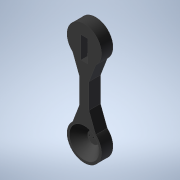
# Autodesk Inventor part: 1st-arm
Saved by Autodesk Inventor 2022 (Build 260153000, 153)
## iProperties
Created: 2022-02-04
Part Number: 1st-arm
Material: Generic
Document SubType Name: Modeling
Designer: Alexa
Density: 1 g/cm^3
Appearance: Default
Author: Alexa
Autodesk Inventor part; units mm, degrees
ref_plane "YZ Plane" through (0, 0, 0) normal (1, 0, 0) x (0, 1, 0)
ref_plane "XZ Plane" through (0, 0, 0) normal (0, 1, 0) x (-1, 0, 0)
ref_plane "XY Plane" through (0, 0, 0) normal (0, 0, 1) x (1, 0, 0)
sketch "Sketch1" plane through (0, 0, 0) normal (0, 0, 1) x (1, 0, 0)
  circle A0 centre (0, 0) radius 30
  line L0 (0, 0) -> (20, 0)
  line L1 (20, 0) -> (20, 150)
  line L2 (20, 150) -> (0, 150)
  line L3 (0, 150) -> (0, 0)
  line L4 (0, 0) -> (-20, 0)
  line L5 (-20, 0) -> (-20, 150)
  line L6 (-20, 150) -> (0, 150)
  line L7 (0, 150) -> (0, 0)
  circle A1 centre (0, 150) radius 30
  point P0 (20, 127.6393)
  point P1 (-20, 127.6393)
  point P2 (-20, 22.3607)
  point P3 (20, 22.3607)
  dimension "d0" = 60
  dimension "d1" = 20
  dimension "d2" = 150
  dimension "d3" = 20
  dimension "d4" = 60
  constraints: 16 end point, 4 parallel, 2 centre point, 2 coincident, 2 horizontal, 2 perpendicular, 1 point on line
  measures "d0" diameter of A0
  measures "d1" distance of L2.end L1.end
  measures "d2" distance of L1.end L0.end
  measures "d3" distance of L5.end L6.end
  measures "d4" diameter of A1
extrude "Extrusion1" add sketch "Sketch1" along normal blind 20
sketch "Sketch2" plane through (0, 0, 20) normal (0, 0, 1) x (1, 0, 0)
  circle A0 centre (0, 0) radius 10
  dimension "d7" = 20
  constraints: 1 centre point, 1 coincident
  measures "d7" diameter of A0
extrude "Extrusion2" cut sketch "Sketch2" against normal blind 16
sketch "Sketch3" plane through (0, 0, 4) normal (0, 0, 1) x (1, 0, 0)
  circle A0 centre (0, 0) radius 1.5
  circle A1 centre (-7, 0) radius 1.5
  circle A2 centre (7, 0) radius 1.5
  dimension "d10" = 3
  dimension "d11" = 3
  dimension "d12" = 3
  constraints: 3 centre point, 1 coincident
  measures "d10" diameter of A0
  measures "d11" diameter of A1
  measures "d12" diameter of A2
extrude "Extrusion3" cut sketch "Sketch3" against normal blind 25.275
sketch "Sketch4" plane through (0, 0, 20) normal (0, 0, 1) x (1, 0, 0)
  circle A0 centre (0, 150) radius 10
  line L0 (-10, 150) -> (10, 150)
  line L1 (10, 150) -> (10, 110)
  line L2 (10, 110) -> (-10, 110)
  line L3 (-10, 110) -> (-10, 150)
  circle A1 centre (0, 150) radius 6
  line L4 (-6, 150) -> (6, 150)
  line L5 (6, 150) -> (6, 127)
  line L6 (6, 127) -> (-6, 127)
  line L7 (-6, 127) -> (-6, 150)
  line L8 (-6, 150) -> (6, 150)
  line L9 (6, 150) -> (6, 156)
  line L10 (6, 156) -> (-6, 156)
  line L11 (-6, 156) -> (-6, 150)
  point P0 (0, 0)
  dimension "d15" = 20
  dimension "d17" = 12
  dimension "d16" = 40
  dimension "d18" = 23
  constraints: 24 end point, 6 parallel, 3 horizontal, 3 perpendicular, 2 horizontal alignment, 1 coincident, 1 point on line, 4 other
  measures "d16" distance of L0.end L1.end
  measures "d18" distance of L4.end L5.end
extrude "Extrusion4" cut sketch "Sketch4" against normal blind 13 contours L5 L6 L7 A0 | A0 L7 A1 L5 | A1 L0 | L0 A1 | A1 L10 L9 | L11 L10 A1
sketch "Sketch5" plane through (0, 0, 20) normal (0, 0, 1) x (1, 0, 0)
  line L0 (6, 127) -> (-6, 127) projected
  line L1 (-6, 127) -> (6, 127)
  line L2 (6, 127) -> (6, 122.3)
  line L3 (6, 122.3) -> (-6, 122.3)
  line L4 (-6, 122.3) -> (-6, 127)
  line L5 (-6, 156) -> (6, 156) projected
  line L6 (-6, 156) -> (6, 156)
  line L7 (6, 156) -> (6, 160.7)
  line L8 (6, 160.7) -> (-6, 160.7)
  line L9 (-6, 160.7) -> (-6, 156)
  point P0 (0, 0)
  dimension "d21" = 4.7
  dimension "d22" = 4.7
  constraints: 16 end point, 4 parallel, 2 horizontal, 2 perpendicular, 1 point on line
  measures "d21" distance of L1.end L2.end
  measures "d22" distance of L7.end L6.end
extrude "Extrusion5" cut sketch "Sketch5" against normal blind 11.5
sketch "Sketch6" plane through (0, 0, 8.5) normal (0, 0, 1) x (1, 0, 0)
  line L0 (-6, 160.7) -> (6, 160.7) projected
  line L1 (6, 160.7) -> (6, 156) projected
  line L2 (-6, 160.7) -> (6, 160.7)
  line L3 (6, 160.7) -> (6, 158.4)
  line L4 (6, 158.4) -> (-6, 158.4)
  line L5 (-6, 158.4) -> (-6, 160.7)
  circle A0 centre (0, 158.4) radius 1
  line L6 (-6, 122.3) -> (-6, 127) projected
  line L7 (6, 127) -> (6, 122.3) projected
  line L8 (-6, 122.3) -> (6, 122.3)
  line L9 (6, 122.3) -> (6, 124.6)
  line L10 (6, 124.6) -> (-6, 124.6)
  line L11 (-6, 124.6) -> (-6, 122.3)
  circle A1 centre (0, 124.6) radius 1
  point P0 (0, 0)
  dimension "d25" = 2.3
  dimension "d26" = 2
  dimension "d27" = 2.3
  dimension "d28" = 2
  constraints: 16 end point, 4 parallel, 2 centre point, 2 horizontal, 2 midpoint, 2 perpendicular, 2 point on line
  measures "d25" distance of L2.end L3.end
  measures "d26" diameter of A0
  measures "d27" distance of L9.end L8.end
  measures "d28" diameter of A1
extrude "Extrusion6" cut sketch "Sketch6" against normal blind 5 contours A0 L4 | L4 A0 | A1 L10 | L10 A1
sketch "Sketch7" plane through (0, 0, 0) normal (0, 0, -1) x (-1, 0, 0)
  circle A0 centre (0, 150) radius 10
  point P0 (0, 0)
  dimension "d31" = 20
  constraints: 1 centre point
  measures "d31" diameter of A0
extrude "Extrusion7" cut sketch "Sketch7" against normal blind 8
chamfer "Chamfer1" distance 16 angle 45 1 edges at (-10, 0, 20)
sketch "Sketch8" plane through (0, 0, 20) normal (0, 0, 1) x (1, 0, 0)
  arc A0 (20, 127.6393) -> (-20, 127.6393) centre (0, 150) ccw projected
  line L0 (-20, 127.6393) -> (-20, 22.3607) projected
  line L1 (20, 127.6393) -> (-20, 22.3607)
  line L2 (-20, 22.3607) -> (-20, 127.6393)
  line L3 (20, 22.3607) -> (20, 127.6393) projected
  line L4 (-20, 127.6393) -> (20, 22.3607)
  line L5 (20, 127.6393) -> (20, 22.3607)
  line L6 (0, 75) -> (8.2239, 75)
  line L7 (8.2239, 75) -> (8.2239, 53.3549)
  line L8 (8.2239, 53.3549) -> (0, 53.3549)
  line L9 (0, 53.3549) -> (0, 75)
  line L10 (0, 75) -> (-8.2239, 75)
  line L11 (-8.2239, 75) -> (-8.2239, 53.3549)
  line L12 (-8.2239, 53.3549) -> (0, 53.3549)
  line L13 (0, 53.3549) -> (0, 75)
  line L14 (8.2239, 75) -> (-8.2239, 75)
  line L15 (-8.2239, 75) -> (-8.2239, 96.6451)
  line L16 (-8.2239, 96.6451) -> (8.2239, 96.6451)
  line L17 (8.2239, 96.6451) -> (8.2239, 75)
  point P0 (0, 0)
  constraints: 32 end point, 6 parallel, 5 point on line, 3 horizontal, 3 perpendicular, 1 midpoint, 1 vertical
extrude "Extrusion8" cut sketch "Sketch8" against normal blind 64.1375 contours L3 L4 L7 L17 L1 | L4 L15 L11 L1 L0
body "Solid1"
